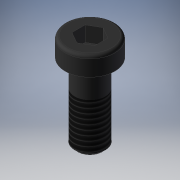
# Autodesk Inventor part: Zylinderschraube DIN 6912 M8x20
Saved by Autodesk Inventor 2019 (Build 230136000, 136)
## iProperties
Created: 2023-08-22
Part Number: Zylinderschraube DIN 6912 M8x20
Material: Generic
Catalog Web Link: www.cadenas.de
Description: DIN 6912 M8x20 NIKO-Hexagon socket head cap screws with low head
Vendor: ROBOTUNITS
Document SubType Name: Modeling
Designer: psAdmin
Manufacturer: ROBOTUNITS
Mass: 1.53189 g
Surface Area: 10.291 cm^2
Volume: 1.53189 cm^3
Density: 1 g/cm^3
Appearance: PSOLRGB-175-175-175
Category: PARTsolutions
Company: ROBOTUNITS
Title: Zylinderschraube DIN 6912 M8x20
Author: Cadenas PARTsolutions
Comments: Hexagon socket head cap screws with low head
PSOL_IDENT_0: {$CADENAS_DATA/23d-libs/robotunits/profil_und_verbindungstechnik/verbindungstechnik_raster_40/parts/
PSOL_IDENT_1: din6912_m8x20niko.prj},215 {VTYP=3D},{NB=Zylinderschraube DIN 6912 M8x20},{LINA=Zylinderschraube DIN
PSOL_IDENT_2: 6912 M8x20},{NN=DIN 6912 M8x20 NIKO},{DATE=25.04.2023 11:25:32},{GEOMDATE=08.04.2014 11:44:00},{VER
PSOL_IDENT_3: SION=},{LINEID=10},{WBVAR=},{WBNUMERIC=}  {NB=Zylinderschraube DIN 6912 M8x20},{LINA=Zylinderschraub
PSOL_IDENT_4: e DIN 6912 M8x20},{KT=DUMMY},{D=8.000},{L=20.000}
NB: Zylinderschraube DIN 6912 M8x20
NN: DIN 6912 M8x20 NIKO
NT: Hexagon socket head cap screws with low head
NBSYN: Zylinderschraube DIN 6912 M8x20
LINA: Zylinderschraube DIN 6912 M8x20
CATALOG: Robotunits
D: 8
L: 20
SUPPLIER: ROBOTUNITS
ARTICLENO: Zylinderschraube DIN 6912 M8x20
BOMINFO: Zylinderschraube DIN 6912 M8x20
CREATOR: CADENAS GmbH
Autodesk Inventor part; units mm, degrees
ref_plane "YZ Plane" through (0, 0, 0) normal (1, 0, 0) x (0, 1, 0)
ref_plane "XZ Plane" through (0, 0, 0) normal (0, 1, 0) x (-1, 0, 0)
ref_plane "XY Plane" through (0, 0, 0) normal (0, 0, 1) x (1, 0, 0)
sketch "Sketch_1" plane through (0, 0, 0) normal (0, 0, 1) x (1, 0, 0)
  line L0 (0, -50) -> (0, 50)
  line L1 (0, 0) -> (5.7, 0)
  arc A0 (6.5, -0.8) -> (5.7, 0) centre (5.7, -0.8) ccw
  line L2 (6.5, -0.8) -> (6.5, -5)
  line L3 (6.5, -5) -> (4, -5)
  line L4 (4, -5) -> (4, -24.233)
  line L5 (4, -24.233) -> (3.233, -25)
  line L6 (3.233, -25) -> (0, -25)
  line L7 (0, -25) -> (0, 0)
  constraints: 16 end point, 2 point on circle, 1 centre point
revolve "Revolution1" add sketch "Sketch_1" angle 360 about axis through (0, -50, 0) along (0, -1, 0)
thread "Thread1" size "M8x1.25" class "6g" standard "ISO Metric profile" length 12.233
sketch "Sketch_2" plane through (0, 0, 0) normal (0, 1, 0) x (-1, 0, 0)
  line L0 (3, 1.7321) -> (0, 3.4641)
  line L1 (0, 3.4641) -> (-3, 1.7321)
  line L2 (-3, 1.7321) -> (-3, -1.7321)
  line L3 (-3, -1.7321) -> (0, -3.4641)
  line L4 (0, -3.4641) -> (3, -1.7321)
  line L5 (3, -1.7321) -> (3, 1.7321)
  constraints: 12 end point
extrude "Extrusion1" cut sketch "Sketch_2" against normal blind 4
ref_plane "p1_XY" through (0, -5, 0) normal (0, -1, 0) x (1, 0, 0)
ref_plane "p1_YZ" through (0, -5, 0) normal (1, 0, 0) x (0, 0, 1)
ref_plane "p1_ZX" through (0, -5, 0) normal (0, 0, 1) x (0, -1, 0)
body "Solid1"
